Theseus_V3_rev4 (Autodesk Fusion 360 design; units mm, degrees)
Autodesk Fusion 360 part; units mm, degrees
note: some values were not read from the file. Chosen so that the rebuilt part matches the saved one: which bodies a step acts on; a direction. Set by a fixed rule: which sketch regions a step uses.
(part 1 of 5)
sketch "Tub shell sketch" plane through (0, 0, 0) normal (0, 0, 1) x (1, 0, 0) in component "Tub"
  circle A0 centre (0, 0) radius 105
extrude "Tub shell" add sketch "Tub shell sketch" along normal blind 52 from surface at 35 makes body 1 in component "Tub"
sketch "Cavity sketch" plane through (0, 0, 0) normal (0, 0, 1) x (1, 0, 0) in component "Tub"
  circle A0 centre (0, 0) radius 103
extrude "Cavity" cut sketch "Cavity sketch" along normal blind 53 from surface at 39 bodies 1 in component "Tub"
sketch "Rear chamfer sketch" plane through (0, 0, 0) normal (0, 1, 0) x (1, 0, 0) in component "Tub"
  line L0 (-65, -35) -> (-112, -56.15)
  line L1 (-112, -56.15) -> (-112, -29)
  line L2 (-112, -29) -> (-65, -29)
  line L3 (-65, -29) -> (-65, -35)
extrude "Rear chamfer" cut sketch "Rear chamfer sketch" along normal blind 220 from surface at -110 bodies 1 in component "Tub"
sketch "Wheel opening and arch L sketch" plane through (0, 0, 0) normal (0, 0, 1) x (1, 0, 0) in component "Tub"
  line L0 (-44, 69) -> (44, 69)
  line L1 (44, 69) -> (44, 108)
  line L2 (44, 108) -> (-44, 108)
  line L3 (-44, 108) -> (-44, 69)
extrude "Wheel opening and arch L" cut sketch "Wheel opening and arch L sketch" along normal blind 49 from surface at 34 bodies 1 in component "Tub"
sketch "Camera notch L sketch" plane through (0, 0, 0) normal (0, 0, 1) x (1, 0, 0) in component "Tub"
  line L0 (-11.9288, 69) -> (18.0712, 69)
  line L1 (18.0712, 69) -> (18.0712, 108)
  line L2 (18.0712, 108) -> (-11.9288, 108)
  line L3 (-11.9288, 108) -> (-11.9288, 69)
extrude "Camera notch L" cut sketch "Camera notch L sketch" along normal blind 6 from surface at 82 bodies 1 in component "Tub"
sketch "Motor seat L sketch" plane through (0, 0, 0) normal (0, 1, 0) x (1, 0, 0) in component "Tub"
  circle A0 centre (0, -40) radius 10.15
extrude "Motor seat L" cut sketch "Motor seat L sketch" along normal blind 51.5 from surface at 13 bodies 1 in component "Tub"
sketch "Shaft notch L sketch" plane through (0, 0, 0) normal (0, 1, 0) x (1, 0, 0) in component "Tub"
  line L0 (-3, -34.5) -> (3, -34.5)
  line L1 (3, -34.5) -> (3, -44.5)
  line L2 (3, -44.5) -> (-3, -44.5)
  line L3 (-3, -44.5) -> (-3, -34.5)
extrude "Shaft notch L" cut sketch "Shaft notch L sketch" along normal blind 4.5 from surface at 64.5 bodies 1 in component "Tub"
sketch "Plate slot L sketch" plane through (0, 0, 0) normal (0, 0, 1) x (1, 0, 0) in component "Tub"
  line L0 (-16, 60.5) -> (24.5, 60.5)
  line L1 (24.5, 60.5) -> (24.5, 64.5)
  line L2 (24.5, 64.5) -> (-16, 64.5)
  line L3 (-16, 64.5) -> (-16, 60.5)
extrude "Plate slot L" cut sketch "Plate slot L sketch" along normal blind 5 from surface at 34.5 bodies 1 in component "Tub"
sketch "Wheel opening and arch R sketch" plane through (0, 0, 0) normal (0, 0, 1) x (1, 0, 0) in component "Tub"
  line L0 (-44, -108) -> (44, -108)
  line L1 (44, -108) -> (44, -69)
  line L2 (44, -69) -> (-44, -69)
  line L3 (-44, -69) -> (-44, -108)
extrude "Wheel opening and arch R" cut sketch "Wheel opening and arch R sketch" along normal blind 49 from surface at 34 bodies 1 in component "Tub"
sketch "Camera notch R sketch" plane through (0, 0, 0) normal (0, 0, 1) x (1, 0, 0) in component "Tub"
  line L0 (-11.9288, -108) -> (18.0712, -108)
  line L1 (18.0712, -108) -> (18.0712, -69)
  line L2 (18.0712, -69) -> (-11.9288, -69)
  line L3 (-11.9288, -69) -> (-11.9288, -108)
extrude "Camera notch R" cut sketch "Camera notch R sketch" along normal blind 6 from surface at 82 bodies 1 in component "Tub"
sketch "Motor seat R sketch" plane through (0, 0, 0) normal (0, 1, 0) x (1, 0, 0) in component "Tub"
  circle A0 centre (0, -40) radius 10.15
extrude "Motor seat R" cut sketch "Motor seat R sketch" along normal blind 51.5 from surface at -64.5 bodies 1 in component "Tub"
sketch "Shaft notch R sketch" plane through (0, 0, 0) normal (0, 1, 0) x (1, 0, 0) in component "Tub"
  line L0 (-3, -34.5) -> (3, -34.5)
  line L1 (3, -34.5) -> (3, -44.5)
  line L2 (3, -44.5) -> (-3, -44.5)
  line L3 (-3, -44.5) -> (-3, -34.5)
extrude "Shaft notch R" cut sketch "Shaft notch R sketch" along normal blind 4.5 from surface at -69 bodies 1 in component "Tub"
sketch "Plate slot R sketch" plane through (0, 0, 0) normal (0, 0, 1) x (1, 0, 0) in component "Tub"
  line L0 (-16, -64.5) -> (24.5, -64.5)
  line L1 (24.5, -64.5) -> (24.5, -60.5)
  line L2 (24.5, -60.5) -> (-16, -60.5)
  line L3 (-16, -60.5) -> (-16, -64.5)
extrude "Plate slot R" cut sketch "Plate slot R sketch" along normal blind 5 from surface at 34.5 bodies 1 in component "Tub"
sketch "Omni wheel opening sketch" plane through (0, 0, 0) normal (0, 0, 1) x (1, 0, 0) in component "Tub"
  line L0 (36.5, -11.3) -> (101, -11.3)
  line L1 (101, -11.3) -> (101, 17.3)
  line L2 (101, 17.3) -> (36.5, 17.3)
  line L3 (36.5, 17.3) -> (36.5, -11.3)
extrude "Omni wheel opening" cut sketch "Omni wheel opening sketch" along normal blind 6 from surface at 34 bodies 1 in component "Tub"
sketch "Omni arm corridor sketch" plane through (0, 0, 0) normal (0, 0, 1) x (1, 0, 0) in component "Tub"
  line L0 (16.5928, 7.5) -> (80, 7.5)
  line L1 (80, 7.5) -> (80, 21)
  line L2 (80, 21) -> (16.5928, 21)
  line L3 (16.5928, 21) -> (16.5928, 7.5)
extrude "Omni arm corridor" cut sketch "Omni arm corridor sketch" along normal blind 6 from surface at 34 bodies 1 in component "Tub"
sketch "Omni pillar sketch" plane through (0, 0, 0) normal (0, 0, 1) x (1, 0, 0) in component "Tub"
  line L0 (17.7928, 3.5) -> (35.5, 3.5)
  line L1 (35.5, 3.5) -> (35.5, 7.5)
  line L2 (35.5, 7.5) -> (17.7928, 7.5)
  line L3 (17.7928, 7.5) -> (17.7928, 3.5)
extrude "Omni pillar" add sketch "Omni pillar sketch" along normal blind 11 from surface at 38.5 bodies 1 in component "Tub"
sketch "Omni pillar tail sketch" plane through (0, 0, 0) normal (0, 0, 1) x (1, 0, 0) in component "Tub"
  line L0 (9.8928, 3.5) -> (17.7928, 3.5)
  line L1 (17.7928, 3.5) -> (17.7928, 12)
  line L2 (17.7928, 12) -> (9.8928, 12)
  line L3 (9.8928, 12) -> (9.8928, 3.5)
extrude "Omni pillar tail" add sketch "Omni pillar tail sketch" along normal blind 5.5 from surface at 38.5 bodies 1 in component "Tub"
sketch "Omni ear sketch" plane through (0, 0, 0) normal (0, 0, 1) x (1, 0, 0) in component "Tub"
  line L0 (19.0928, 21) -> (36.5, 21)
  line L1 (36.5, 21) -> (36.5, 29.8)
  line L2 (36.5, 29.8) -> (19.0928, 29.8)
  line L3 (19.0928, 29.8) -> (19.0928, 21)
extrude "Omni ear" add sketch "Omni ear sketch" along normal blind 8.5 from surface at 38.5 bodies 1 in component "Tub"
sketch "Pivot hole pillar sketch" plane through (0, 0, 0) normal (0, 1, 0) x (1, 0, 0) in component "Tub"
  circle A0 centre (24.0928, -42) radius 1.6
extrude "Pivot hole pillar" cut sketch "Pivot hole pillar sketch" along normal blind 6 from surface at 2.5 bodies 1 in component "Tub"
sketch "Pivot thread hole ear sketch" plane through (0, 0, 0) normal (0, 1, 0) x (1, 0, 0) in component "Tub"
  circle A0 centre (24.0928, -42) radius 1.5
extrude "Pivot thread hole ear" cut sketch "Pivot thread hole ear sketch" along normal blind 8.1 from surface at 20.5 bodies 1 in component "Tub"
sketch "Stop hole pillar sketch" plane through (0, 0, 0) normal (0, 1, 0) x (1, 0, 0) in component "Tub"
  circle A0 centre (32.0923, -42.0904) radius 1.6
extrude "Stop hole pillar" cut sketch "Stop hole pillar sketch" along normal blind 6 from surface at 2.5 bodies 1 in component "Tub"
sketch "Stop thread hole ear sketch" plane through (0, 0, 0) normal (0, 1, 0) x (1, 0, 0) in component "Tub"
  circle A0 centre (32.0923, -42.0904) radius 1.5
extrude "Stop thread hole ear" cut sketch "Stop thread hole ear sketch" along normal blind 8.1 from surface at 20.5 bodies 1 in component "Tub"
sketch "Adjuster hole tail sketch" plane through (0, 0, 0) normal (0, 0, 1) x (1, 0, 0) in component "Tub"
  circle A0 centre (14.0928, 8.8) radius 1.5
extrude "Adjuster hole tail" cut sketch "Adjuster hole tail sketch" along normal blind 6.8 from surface at 38.2 bodies 1 in component "Tub"
sketch "Floor port FP hole sketch" plane through (0, 0, 0) normal (0, 0, 1) x (1, 0, 0) in component "Tub"
  line L0 (64.35, 24.35) -> (85.65, 24.35)
  line L1 (85.65, 24.35) -> (85.65, 45.65)
  line L2 (85.65, 45.65) -> (64.35, 45.65)
  line L3 (64.35, 45.65) -> (64.35, 24.35)
extrude "Floor port FP hole" cut sketch "Floor port FP hole sketch" along normal blind 6 from surface at 34 bodies 1 in component "Tub"
sketch "Silver module SM hole sketch" plane through (0, 0, 0) normal (0, 0, 1) x (1, 0, 0) in component "Tub"
  line L0 (64.5, -38.5) -> (85.5, -38.5)
  line L1 (85.5, -38.5) -> (85.5, -15.5)
  line L2 (85.5, -15.5) -> (64.5, -15.5)
  line L3 (64.5, -15.5) -> (64.5, -38.5)
extrude "Silver module SM hole" cut sketch "Silver module SM hole sketch" along normal blind 6 from surface at 34 bodies 1 in component "Tub"
sketch "Chute hole tool B left sketch" plane through (0, 0, 0) normal (0, 0, 1) x (1, 0, 0) in component "Tub"
  line L0 (-11.5, -10) -> (11.5, -10)
  line L1 (11.5, -10) -> (11.5, 13)
  line L2 (11.5, 13) -> (-11.5, 13)
  line L3 (-11.5, 13) -> (-11.5, -10)
extrude "Chute hole tool B left" add sketch "Chute hole tool B left sketch" along normal blind 79.2151 separate body makes body 2 in component "Tub"
move_body "Move1" bodies 2 to x (-0.977496, -0.210954, 0) y (-0.112564, 0.521586, 0.845741) z (-0.178413, 0.826708, -0.533594) at (-47.2943, 27.2943, 79.5) in component "Tub"
combine "Combine1" operation cut target body 1 tool bodies 2 in component "Tub"
sketch "Chute hole tool A right sketch" plane through (0, 0, 0) normal (0, 0, 1) x (1, 0, 0) in component "Tub"
  line L0 (-11.5, -10) -> (11.5, -10)
  line L1 (11.5, -10) -> (11.5, 13)
  line L2 (11.5, 13) -> (-11.5, 13)
  line L3 (-11.5, 13) -> (-11.5, -10)
extrude "Chute hole tool A right" add sketch "Chute hole tool A right sketch" along normal blind 79.2151 separate body makes body 3 in component "Tub"
move_body "Move2" bodies 3 to x (0.977496, -0.210954, 0) y (-0.112564, -0.521586, 0.845741) z (-0.178413, -0.826708, -0.533594) at (-47.2943, -27.2943, 79.5) in component "Tub"
combine "Combine2" operation cut target body 1 tool bodies 3 in component "Tub"
sketch "Bumper recess L sketch" plane through (0, 0, 0) normal (0, 0, 1) x (1, 0, 0) in component "Tub"
  arc A0 (106.949, 15.0307) -> (50.7029, 95.3583) centre (0, 0) ccw
  line L0 (50.7029, 95.3583) -> (48.5903, 91.3851)
  arc A1 (102.4927, 14.4044) -> (48.5903, 91.3851) centre (0, 0) ccw
  line L1 (102.4927, 14.4044) -> (106.949, 15.0307)
extrude "Bumper recess L" cut sketch "Bumper recess L sketch" along normal blind 25 from surface at 40 bodies 1 in component "Tub"
sketch "Bumper recess wall L sketch" plane through (0, 0, 0) normal (0, 0, 1) x (1, 0, 0) in component "Tub"
  arc A0 (102.1957, 14.3627) -> (48.4495, 91.1202) centre (0, 0) ccw
  line L0 (48.4495, 91.1202) -> (47.6514, 89.6192)
  arc A1 (100.5122, 14.1261) -> (47.6514, 89.6192) centre (0, 0) ccw
  line L1 (100.5122, 14.1261) -> (102.1957, 14.3627)
extrude "Bumper recess wall L" add sketch "Bumper recess wall L sketch" along normal blind 27 from surface at 39 bodies 1 in component "Tub"
sketch "Bumper switch pocket L sketch" plane through (0, 0, 0) normal (0, 0, 1) x (1, 0, 0) in component "Tub"
  line L0 (98.18, 21.6448) -> (101.576, 22.4916)
  line L1 (101.576, 22.4916) -> (100.2455, 27.8282)
  line L2 (100.2455, 27.8282) -> (96.8494, 26.9815)
  line L3 (96.8494, 26.9815) -> (98.18, 21.6448)
extrude "Bumper switch pocket L" cut sketch "Bumper switch pocket L sketch" along normal blind 12 from surface at 46.5 bodies 1 in component "Tub"
sketch "Bumper recess R sketch" plane through (0, 0, 0) normal (0, 0, 1) x (1, 0, 0) in component "Tub"
  arc A0 (50.7029, -95.3583) -> (106.949, -15.0307) centre (0, 0) ccw
  line L0 (106.949, -15.0307) -> (102.4927, -14.4044)
  arc A1 (48.5903, -91.3851) -> (102.4927, -14.4044) centre (0, 0) ccw
  line L1 (48.5903, -91.3851) -> (50.7029, -95.3583)
extrude "Bumper recess R" cut sketch "Bumper recess R sketch" along normal blind 25 from surface at 40 bodies 1 in component "Tub"
sketch "Bumper recess wall R sketch" plane through (0, 0, 0) normal (0, 0, 1) x (1, 0, 0) in component "Tub"
  arc A0 (48.4495, -91.1202) -> (102.1957, -14.3627) centre (0, 0) ccw
  line L0 (102.1957, -14.3627) -> (100.5122, -14.1261)
  arc A1 (47.6514, -89.6192) -> (100.5122, -14.1261) centre (0, 0) ccw
  line L1 (47.6514, -89.6192) -> (48.4495, -91.1202)
extrude "Bumper recess wall R" add sketch "Bumper recess wall R sketch" along normal blind 27 from surface at 39 bodies 1 in component "Tub"
sketch "Bumper switch pocket R sketch" plane through (0, 0, 0) normal (0, 0, 1) x (1, 0, 0) in component "Tub"
  line L0 (96.8494, -26.9815) -> (100.2455, -27.8282)
  line L1 (100.2455, -27.8282) -> (101.576, -22.4916)
  line L2 (101.576, -22.4916) -> (98.18, -21.6448)
  line L3 (98.18, -21.6448) -> (96.8494, -26.9815)
extrude "Bumper switch pocket R" cut sketch "Bumper switch pocket R sketch" along normal blind 12 from surface at 46.5 bodies 1 in component "Tub"
sketch "Insert boss +12 sketch" plane through (0, 0, 0) normal (0, 0, 1) x (1, 0, 0) in component "Tub"
  circle A0 centre (95.3694, 20.2714) radius 6
  line L0 (96.4089, 15.3807) -> (102.7669, 16.7321)
  line L1 (102.7669, 16.7321) -> (100.6878, 26.5136)
  line L2 (100.6878, 26.5136) -> (94.3298, 25.1621)
  line L3 (94.3298, 25.1621) -> (96.4089, 15.3807)
extrude "Insert boss +12" add sketch "Insert boss +12 sketch" along normal blind 10 from surface at 77 bodies 1 in component "Tub"
sketch "Insert boss +60 sketch" plane through (0, 0, 0) normal (0, 0, 1) x (1, 0, 0) in component "Tub"
  circle A0 centre (48.75, 84.4375) radius 6
  line L0 (53.0801, 81.9375) -> (56.3301, 87.5666)
  line L1 (56.3301, 87.5666) -> (47.6699, 92.5666)
  line L2 (47.6699, 92.5666) -> (44.4199, 86.9375)
  line L3 (44.4199, 86.9375) -> (53.0801, 81.9375)
extrude "Insert boss +60" add sketch "Insert boss +60 sketch" along normal blind 10 from surface at 77 bodies 1 in component "Tub"
sketch "Insert boss +118 sketch" plane through (0, 0, 0) normal (0, 0, 1) x (1, 0, 0) in component "Tub"
  circle A0 centre (-45.7735, 86.0874) radius 6
  line L0 (-41.3587, 88.4347) -> (-44.4103, 94.1739)
  line L1 (-44.4103, 94.1739) -> (-53.2398, 89.4792)
  line L2 (-53.2398, 89.4792) -> (-50.1882, 83.74)
  line L3 (-50.1882, 83.74) -> (-41.3587, 88.4347)
extrude "Insert boss +118" add sketch "Insert boss +118 sketch" along normal blind 10 from surface at 77 bodies 1 in component "Tub"
sketch "Insert boss -12 sketch" plane through (0, 0, 0) normal (0, 0, 1) x (1, 0, 0) in component "Tub"
  circle A0 centre (95.3694, -20.2714) radius 6
  line L0 (94.3298, -25.1621) -> (100.6878, -26.5136)
  line L1 (100.6878, -26.5136) -> (102.7669, -16.7321)
  line L2 (102.7669, -16.7321) -> (96.4089, -15.3807)
  line L3 (96.4089, -15.3807) -> (94.3298, -25.1621)
extrude "Insert boss -12" add sketch "Insert boss -12 sketch" along normal blind 10 from surface at 77 bodies 1 in component "Tub"
sketch "Insert boss -60 sketch" plane through (0, 0, 0) normal (0, 0, 1) x (1, 0, 0) in component "Tub"
  circle A0 centre (48.75, -84.4375) radius 6
  line L0 (44.4199, -86.9375) -> (47.6699, -92.5666)
  line L1 (47.6699, -92.5666) -> (56.3301, -87.5666)
  line L2 (56.3301, -87.5666) -> (53.0801, -81.9375)
  line L3 (53.0801, -81.9375) -> (44.4199, -86.9375)
extrude "Insert boss -60" add sketch "Insert boss -60 sketch" along normal blind 10 from surface at 77 bodies 1 in component "Tub"
sketch "Insert boss -118 sketch" plane through (0, 0, 0) normal (0, 0, 1) x (1, 0, 0) in component "Tub"
  circle A0 centre (-45.7735, -86.0874) radius 6
  line L0 (-50.1882, -83.74) -> (-53.2398, -89.4792)
  line L1 (-53.2398, -89.4792) -> (-44.4103, -94.1739)
  line L2 (-44.4103, -94.1739) -> (-41.3587, -88.4347)
  line L3 (-41.3587, -88.4347) -> (-50.1882, -83.74)
extrude "Insert boss -118" add sketch "Insert boss -118 sketch" along normal blind 10 from surface at 77 bodies 1 in component "Tub"
sketch "Cradle web rear L sketch" plane through (0, 0, 0) normal (0, 1, 0) x (1, 0, 0) in component "Tub"
  line L0 (-16, -38.5) -> (-3, -38.5)
  line L1 (-3, -38.5) -> (-3, -52)
  line L2 (-3, -52) -> (-16, -52)
  line L3 (-16, -52) -> (-16, -38.5)
extrude "Cradle web rear L" add sketch "Cradle web rear L sketch" along normal blind 2.5 from surface at 64.5 bodies 1 in component "Tub"
sketch "Cradle web front L sketch" plane through (0, 0, 0) normal (0, 1, 0) x (1, 0, 0) in component "Tub"
  line L0 (3, -38.5) -> (27.5, -38.5)
  line L1 (27.5, -38.5) -> (27.5, -52)
  line L2 (27.5, -52) -> (3, -52)
  line L3 (3, -52) -> (3, -38.5)
extrude "Cradle web front L" add sketch "Cradle web front L sketch" along normal blind 2.5 from surface at 64.5 bodies 1 in component "Tub"
sketch "Cradle ledge front L sketch" plane through (0, 0, 0) normal (0, 1, 0) x (1, 0, 0) in component "Tub"
  line L0 (10.6, -38.5) -> (27.5, -38.5)
  line L1 (27.5, -38.5) -> (27.5, -49)
  line L2 (27.5, -49) -> (10.6, -49)
  line L3 (10.6, -49) -> (10.6, -38.5)
extrude "Cradle ledge front L" add sketch "Cradle ledge front L sketch" along normal blind 4 from surface at 56.5 bodies 1 in component "Tub"
sketch "Cradle ledge rear L sketch" plane through (0, 0, 0) normal (0, 1, 0) x (1, 0, 0) in component "Tub"
  line L0 (-16, -38.5) -> (-10.6, -38.5)
  line L1 (-10.6, -38.5) -> (-10.6, -49)
  line L2 (-10.6, -49) -> (-16, -49)
  line L3 (-16, -49) -> (-16, -38.5)
extrude "Cradle ledge rear L" add sketch "Cradle ledge rear L sketch" along normal blind 4 from surface at 56.5 bodies 1 in component "Tub"
sketch "Cradle prong front L sketch" plane through (0, 0, 0) normal (0, 1, 0) x (1, 0, 0) in component "Tub"
  line L0 (13, -38.5) -> (13, -48)
  line L1 (13, -48) -> (8, -48)
  line L2 (8, -48) -> (7.8607, -46.5)
  line L3 (7.8607, -46.5) -> (8.544, -45.5714)
  line L4 (8.544, -45.5714) -> (9.0821, -44.6429)
  line L5 (9.0821, -44.6429) -> (9.4997, -43.7143)
  line L6 (9.4997, -43.7143) -> (9.8122, -42.7857)
  line L7 (9.8122, -42.7857) -> (10.0295, -41.8571)
  line L8 (10.0295, -41.8571) -> (10.1576, -40.9286)
  line L9 (10.1576, -40.9286) -> (10.2, -40)
  line L10 (10.2, -40) -> (10.6, -38.5)
  line L11 (10.6, -38.5) -> (13, -38.5)
extrude "Cradle prong front L" add sketch "Cradle prong front L sketch" along normal blind 32 from surface at 28.5 separate body makes body 4 in component "Tub"
sketch "Cradle prong rear L sketch" plane through (0, 0, 0) normal (0, 1, 0) x (1, 0, 0) in component "Tub"
  line L0 (-13, -38.5) -> (-13, -48)
  line L1 (-13, -48) -> (-8, -48)
  line L2 (-8, -48) -> (-7.8607, -46.5)
  line L3 (-7.8607, -46.5) -> (-8.544, -45.5714)
  line L4 (-8.544, -45.5714) -> (-9.0821, -44.6429)
  line L5 (-9.0821, -44.6429) -> (-9.4997, -43.7143)
  line L6 (-9.4997, -43.7143) -> (-9.8122, -42.7857)
  line L7 (-9.8122, -42.7857) -> (-10.0295, -41.8571)
  line L8 (-10.0295, -41.8571) -> (-10.1576, -40.9286)
  line L9 (-10.1576, -40.9286) -> (-10.2, -40)
  line L10 (-10.2, -40) -> (-10.6, -38.5)
  line L11 (-10.6, -38.5) -> (-13, -38.5)
extrude "Cradle prong rear L" add sketch "Cradle prong rear L sketch" along normal blind 32 from surface at 28.5 separate body makes body 5 in component "Tub"
sketch "Cradle web rear R sketch" plane through (0, 0, 0) normal (0, 1, 0) x (1, 0, 0) in component "Tub"
  line L0 (-16, -38.5) -> (-3, -38.5)
  line L1 (-3, -38.5) -> (-3, -52)
  line L2 (-3, -52) -> (-16, -52)
  line L3 (-16, -52) -> (-16, -38.5)
extrude "Cradle web rear R" add sketch "Cradle web rear R sketch" along normal blind 2.5 from surface at -67 bodies 1 in component "Tub"
sketch "Cradle web front R sketch" plane through (0, 0, 0) normal (0, 1, 0) x (1, 0, 0) in component "Tub"
  line L0 (3, -38.5) -> (27.5, -38.5)
  line L1 (27.5, -38.5) -> (27.5, -52)
  line L2 (27.5, -52) -> (3, -52)
  line L3 (3, -52) -> (3, -38.5)
extrude "Cradle web front R" add sketch "Cradle web front R sketch" along normal blind 2.5 from surface at -67 bodies 1 in component "Tub"
sketch "Cradle ledge front R sketch" plane through (0, 0, 0) normal (0, 1, 0) x (1, 0, 0) in component "Tub"
  line L0 (10.6, -38.5) -> (27.5, -38.5)
  line L1 (27.5, -38.5) -> (27.5, -49)
  line L2 (27.5, -49) -> (10.6, -49)
  line L3 (10.6, -49) -> (10.6, -38.5)
extrude "Cradle ledge front R" add sketch "Cradle ledge front R sketch" along normal blind 4 from surface at -60.5 bodies 1 in component "Tub"
sketch "Cradle ledge rear R sketch" plane through (0, 0, 0) normal (0, 1, 0) x (1, 0, 0) in component "Tub"
  line L0 (-16, -38.5) -> (-10.6, -38.5)
  line L1 (-10.6, -38.5) -> (-10.6, -49)
  line L2 (-10.6, -49) -> (-16, -49)
  line L3 (-16, -49) -> (-16, -38.5)
extrude "Cradle ledge rear R" add sketch "Cradle ledge rear R sketch" along normal blind 4 from surface at -60.5 bodies 1 in component "Tub"
sketch "Cradle prong front R sketch" plane through (0, 0, 0) normal (0, 1, 0) x (1, 0, 0) in component "Tub"
  line L0 (13, -38.5) -> (13, -48)
  line L1 (13, -48) -> (8, -48)
  line L2 (8, -48) -> (7.8607, -46.5)
  line L3 (7.8607, -46.5) -> (8.544, -45.5714)
  line L4 (8.544, -45.5714) -> (9.0821, -44.6429)
  line L5 (9.0821, -44.6429) -> (9.4997, -43.7143)
  line L6 (9.4997, -43.7143) -> (9.8122, -42.7857)
  line L7 (9.8122, -42.7857) -> (10.0295, -41.8571)
  line L8 (10.0295, -41.8571) -> (10.1576, -40.9286)
  line L9 (10.1576, -40.9286) -> (10.2, -40)
  line L10 (10.2, -40) -> (10.6, -38.5)
  line L11 (10.6, -38.5) -> (13, -38.5)
extrude "Cradle prong front R" add sketch "Cradle prong front R sketch" along normal blind 32 from surface at -60.5 separate body makes body 6 in component "Tub"
sketch "Cradle prong rear R sketch" plane through (0, 0, 0) normal (0, 1, 0) x (1, 0, 0) in component "Tub"
  line L0 (-13, -38.5) -> (-13, -48)
  line L1 (-13, -48) -> (-8, -48)
  line L2 (-8, -48) -> (-7.8607, -46.5)
  line L3 (-7.8607, -46.5) -> (-8.544, -45.5714)
  line L4 (-8.544, -45.5714) -> (-9.0821, -44.6429)
  line L5 (-9.0821, -44.6429) -> (-9.4997, -43.7143)
  line L6 (-9.4997, -43.7143) -> (-9.8122, -42.7857)
  line L7 (-9.8122, -42.7857) -> (-10.0295, -41.8571)
  line L8 (-10.0295, -41.8571) -> (-10.1576, -40.9286)
  line L9 (-10.1576, -40.9286) -> (-10.2, -40)
  line L10 (-10.2, -40) -> (-10.6, -38.5)
  line L11 (-10.6, -38.5) -> (-13, -38.5)
extrude "Cradle prong rear R" add sketch "Cradle prong rear R sketch" along normal blind 32 from surface at -60.5 separate body makes body 7 in component "Tub"
sketch "Tray leg sketch" plane through (0, 0, 0) normal (0, 0, 1) x (1, 0, 0) in component "Tub"
  circle A0 centre (66.4605, 60.5271) radius 3
extrude "Tray leg" add sketch "Tray leg sketch" along normal blind 11 from surface at 38.5 bodies 1 in component "Tub"
sketch "Tray leg sketch (1)" plane through (0, 0, 0) normal (0, 0, 1) x (1, 0, 0) in component "Tub"
  circle A0 centre (49.3095, 31.1019) radius 3
extrude "Tray leg (1)" add sketch "Tray leg sketch (1)" along normal blind 11 from surface at 38.5 bodies 1 in component "Tub"
sketch "Tray leg sketch (2)" plane through (0, 0, 0) normal (0, 0, 1) x (1, 0, 0) in component "Tub"
  circle A0 centre (32.7439, 44.4277) radius 3
extrude "Tray leg (2)" add sketch "Tray leg sketch (2)" along normal blind 11 from surface at 38.5 bodies 1 in component "Tub"
sketch "Battery tray sketch" plane through (0, 0, 0) normal (0, 0, 1) x (1, 0, 0) in component "Tub"
  line L0 (6.7594, 19.0297) -> (77.6656, 31.5324)
  line L1 (77.6656, 31.5324) -> (71.2406, 67.9703)
  line L2 (71.2406, 67.9703) -> (0.3344, 55.4676)
  line L3 (0.3344, 55.4676) -> (6.7594, 19.0297)
extrude "Battery tray" add sketch "Battery tray sketch" along normal blind 2 from surface at 49 bodies 1 in component "Tub"
sketch "Battery stop sketch" plane through (0, 0, 0) normal (0, 0, 1) x (1, 0, 0) in component "Tub"
  line L0 (77.1732, 31.4456) -> (79.1428, 31.7929)
  line L1 (79.1428, 31.7929) -> (72.7178, 68.2308)
  line L2 (72.7178, 68.2308) -> (70.7482, 67.8835)
  line L3 (70.7482, 67.8835) -> (77.1732, 31.4456)
extrude "Battery stop" add sketch "Battery stop sketch" along normal blind 6.5 from surface at 50.5 bodies 1 in component "Tub"
sketch "Battery tray notch sketch" plane through (0, 0, 0) normal (0, 0, 1) x (1, 0, 0) in component "Tub"
  line L0 (-12, 13) -> (12, 13)
  line L1 (12, 13) -> (12, 62)
  line L2 (12, 62) -> (-12, 62)
  line L3 (-12, 62) -> (-12, 13)
extrude "Battery tray notch" cut sketch "Battery tray notch sketch" along normal blind 4 from surface at 48 bodies 1 in component "Tub"
sketch "Insert hole +12 sketch" plane through (0, 0, 0) normal (0, 0, 1) x (1, 0, 0) in component "Tub"
  circle A0 centre (95.3694, 20.2714) radius 2
extrude "Insert hole +12" cut sketch "Insert hole +12 sketch" along normal blind 7 from surface at 81 bodies 1 in component "Tub"
sketch "Insert hole +60 sketch" plane through (0, 0, 0) normal (0, 0, 1) x (1, 0, 0) in component "Tub"
  circle A0 centre (48.75, 84.4375) radius 2
extrude "Insert hole +60" cut sketch "Insert hole +60 sketch" along normal blind 7 from surface at 81 bodies 1 in component "Tub"
sketch "Insert hole +118 sketch" plane through (0, 0, 0) normal (0, 0, 1) x (1, 0, 0) in component "Tub"
  circle A0 centre (-45.7735, 86.0874) radius 2
extrude "Insert hole +118" cut sketch "Insert hole +118 sketch" along normal blind 7 from surface at 81 bodies 1 in component "Tub"
sketch "Insert hole -12 sketch" plane through (0, 0, 0) normal (0, 0, 1) x (1, 0, 0) in component "Tub"
  circle A0 centre (95.3694, -20.2714) radius 2
extrude "Insert hole -12" cut sketch "Insert hole -12 sketch" along normal blind 7 from surface at 81 bodies 1 in component "Tub"
sketch "Insert hole -60 sketch" plane through (0, 0, 0) normal (0, 0, 1) x (1, 0, 0) in component "Tub"
  circle A0 centre (48.75, -84.4375) radius 2
extrude "Insert hole -60" cut sketch "Insert hole -60 sketch" along normal blind 7 from surface at 81 bodies 1 in component "Tub"
sketch "Insert hole -118 sketch" plane through (0, 0, 0) normal (0, 0, 1) x (1, 0, 0) in component "Tub"
  circle A0 centre (-45.7735, -86.0874) radius 2
extrude "Insert hole -118" cut sketch "Insert hole -118 sketch" along normal blind 7 from surface at 81 bodies 1 in component "Tub"
sketch "IMU posts sketch" plane through (0, 0, 0) normal (0, 0, 1) x (1, 0, 0) in component "Tub"
  line L0 (-42.5, 3.5) -> (-37.5, 3.5)
  line L1 (-37.5, 3.5) -> (-37.5, 8.5)
  line L2 (-37.5, 8.5) -> (-42.5, 8.5)
  line L3 (-42.5, 8.5) -> (-42.5, 3.5)
  line L4 (-42.5, -8.5) -> (-37.5, -8.5)
  line L5 (-37.5, -8.5) -> (-37.5, -3.5)
  line L6 (-37.5, -3.5) -> (-42.5, -3.5)
  line L7 (-42.5, -3.5) -> (-42.5, -8.5)
  line L8 (-62.5, 3.5) -> (-57.5, 3.5)
  line L9 (-57.5, 3.5) -> (-57.5, 8.5)
  line L10 (-57.5, 8.5) -> (-62.5, 8.5)
  line L11 (-62.5, 8.5) -> (-62.5, 3.5)
  line L12 (-62.5, -8.5) -> (-57.5, -8.5)
  line L13 (-57.5, -8.5) -> (-57.5, -3.5)
  line L14 (-57.5, -3.5) -> (-62.5, -3.5)
  line L15 (-62.5, -3.5) -> (-62.5, -8.5)
extrude "IMU posts" add sketch "IMU posts sketch" along normal blind 5.5 from surface at 38.5 bodies 1 in component "Tub"
sketch "IMU post pilots sketch" plane through (0, 0, 0) normal (0, 0, 1) x (1, 0, 0) in component "Tub"
  line L0 (-41, 5) -> (-39, 5)
  line L1 (-39, 5) -> (-39, 7)
  line L2 (-39, 7) -> (-41, 7)
  line L3 (-41, 7) -> (-41, 5)
  line L4 (-41, -7) -> (-39, -7)
  line L5 (-39, -7) -> (-39, -5)
  line L6 (-39, -5) -> (-41, -5)
  line L7 (-41, -5) -> (-41, -7)
  line L8 (-61, 5) -> (-59, 5)
  line L9 (-59, 5) -> (-59, 7)
  line L10 (-59, 7) -> (-61, 7)
  line L11 (-61, 7) -> (-61, 5)
  line L12 (-61, -7) -> (-59, -7)
  line L13 (-59, -7) -> (-59, -5)
  line L14 (-59, -5) -> (-61, -5)
  line L15 (-61, -5) -> (-61, -7)
extrude "IMU post pilots" cut sketch "IMU post pilots sketch" along normal blind 5.5 from surface at 39.5 bodies 1 in component "Tub"
sketch "USB-C socket hole sketch" plane through (0, 0, 0) normal (0, 0, 1) x (1, 0, 0) in component "Tub"
  line L0 (87.5938, -46.6617) -> (95.8158, -50.3224)
  line L1 (95.8158, -50.3224) -> (101.5101, -37.5327)
  line L2 (101.5101, -37.5327) -> (93.2882, -33.8721)
  line L3 (93.2882, -33.8721) -> (87.5938, -46.6617)
extrude "USB-C socket hole" cut sketch "USB-C socket hole sketch" along normal blind 8 from surface at 71 bodies 1 in component "Tub"
sketch "Wheel L sketch" plane through (0, 0, 0) normal (0, 1, 0) x (1, 0, 0) in component "Wheel L"
  circle A0 centre (0, -40) radius 40
extrude "Wheel L" add sketch "Wheel L sketch" along normal blind 20 from surface at 70 separate body makes body 8 in component "Wheel L"
sketch "Shaft bore sketch" plane through (0, 0, 0) normal (0, 1, 0) x (1, 0, 0) in component "Wheel L"
  circle A0 centre (0, -40) radius 1.5
extrude "Shaft bore" cut sketch "Shaft bore sketch" along normal blind 22 from surface at 69 bodies 8 in component "Wheel L"
sketch "Encoder L sketch" plane through (0, 0, 0) normal (0, 1, 0) x (1, 0, 0) in component "Motor L"
  circle A0 centre (0, -40) radius 9
extrude "Encoder L" add sketch "Encoder L sketch" along normal blind 3 from surface at 14 separate body makes body 9 in component "Motor L"
sketch "Gearmotor L sketch" plane through (0, 0, 0) normal (0, 1, 0) x (1, 0, 0) in component "Motor L"
  circle A0 centre (0, -40) radius 10
extrude "Gearmotor L" add sketch "Gearmotor L sketch" along normal blind 44 from surface at 17 separate body makes body 10 in component "Motor L"
sketch "Motor shaft L sketch" plane through (0, 0, 0) normal (0, 1, 0) x (1, 0, 0) in component "Motor L"
  circle A0 centre (0, -40) radius 1.5
extrude "Motor shaft L" add sketch "Motor shaft L sketch" along normal blind 19 from surface at 61 separate body makes body 11 in component "Motor L"
sketch "Wheel R sketch" plane through (0, 0, 0) normal (0, 1, 0) x (1, 0, 0) in component "Wheel R"
  circle A0 centre (0, -40) radius 40
extrude "Wheel R" add sketch "Wheel R sketch" along normal blind 20 from surface at -90 separate body makes body 12 in component "Wheel R"
sketch "Shaft bore sketch (2)" plane through (0, 0, 0) normal (0, 1, 0) x (1, 0, 0) in component "Wheel R"
  circle A0 centre (0, -40) radius 1.5
extrude "Shaft bore'" cut sketch "Shaft bore sketch (2)" along normal blind 22 from surface at -91 bodies 12 in component "Wheel R"
sketch "Encoder R sketch" plane through (0, 0, 0) normal (0, 1, 0) x (1, 0, 0) in component "Motor R"
  circle A0 centre (0, -40) radius 9
extrude "Encoder R" add sketch "Encoder R sketch" along normal blind 3 from surface at -17 separate body makes body 13 in component "Motor R"
sketch "Gearmotor R sketch" plane through (0, 0, 0) normal (0, 1, 0) x (1, 0, 0) in component "Motor R"
  circle A0 centre (0, -40) radius 10
extrude "Gearmotor R" add sketch "Gearmotor R sketch" along normal blind 44 from surface at -61 separate body makes body 14 in component "Motor R"
sketch "Motor shaft R sketch" plane through (0, 0, 0) normal (0, 1, 0) x (1, 0, 0) in component "Motor R"
  circle A0 centre (0, -40) radius 1.5
extrude "Motor shaft R" add sketch "Motor shaft R sketch" along normal blind 19 from surface at -80 separate body makes body 15 in component "Motor R"
sketch "Face plate L sketch" plane through (0, 0, 0) normal (0, 1, 0) x (1, 0, 0) in component "Face plate L"
  line L0 (-15.5, -35.5) -> (23.5, -35.5)
  line L1 (23.5, -35.5) -> (23.5, -46)
  line L2 (23.5, -46) -> (15.5, -46)
  line L3 (15.5, -46) -> (15.5, -51)
  line L4 (15.5, -51) -> (-15.5, -51)
  line L5 (-15.5, -51) -> (-15.5, -35.5)
extrude "Face plate L" add sketch "Face plate L sketch" along normal blind 3 from surface at 61 separate body makes body 16 in component "Face plate L"
sketch "Shaft bore sketch (3)" plane through (0, 0, 0) normal (0, 1, 0) x (1, 0, 0) in component "Face plate L"
  circle A0 centre (0, -40) radius 2.2
extrude "Shaft bore''" cut sketch "Shaft bore sketch (3)" along normal blind 5 from surface at 60 bodies 16 in component "Face plate L"
sketch "Face plate R sketch" plane through (0, 0, 0) normal (0, 1, 0) x (1, 0, 0) in component "Face plate R"
  line L0 (-15.5, -35.5) -> (23.5, -35.5)
  line L1 (23.5, -35.5) -> (23.5, -46)
  line L2 (23.5, -46) -> (15.5, -46)
  line L3 (15.5, -46) -> (15.5, -51)
  line L4 (15.5, -51) -> (-15.5, -51)
  line L5 (-15.5, -51) -> (-15.5, -35.5)
extrude "Face plate R" add sketch "Face plate R sketch" along normal blind 3 from surface at -64 separate body makes body 17 in component "Face plate R"
sketch "Shaft bore sketch (4)" plane through (0, 0, 0) normal (0, 1, 0) x (1, 0, 0) in component "Face plate R"
  circle A0 centre (0, -40) radius 2.2
extrude "Shaft bore'''" cut sketch "Shaft bore sketch (4)" along normal blind 5 from surface at -65 bodies 17 in component "Face plate R"
sketch "Omni wheel sketch" plane through (0, 0, 0) normal (0, 1, 0) x (1, 0, 0) in component "Omni wheel"
  circle A0 centre (68.5, -30) radius 30
extrude "Omni wheel" add sketch "Omni wheel sketch" along normal blind 25.6 from surface at -9.8 separate body makes body 18 in component "Omni wheel"
sketch "Wheel bore sketch" plane through (0, 0, 0) normal (0, 1, 0) x (1, 0, 0) in component "Omni wheel"
  circle A0 centre (68.5, -30) radius 6
extrude "Wheel bore" cut sketch "Wheel bore sketch" along normal blind 27.6 from surface at -10.8 bodies 18 in component "Omni wheel"
sketch "Bearing inboard sketch" plane through (0, 0, 0) normal (0, 1, 0) x (1, 0, 0) in component "Omni wheel"
  circle A0 centre (68.5, -30) radius 6
  circle A1 centre (68.5, -30) radius 2
extrude "Bearing inboard" add sketch "Bearing inboard sketch" along normal blind 4 from surface at -4.8 separate body makes body 19 in component "Omni wheel"
sketch "Bearing outboard sketch" plane through (0, 0, 0) normal (0, 1, 0) x (1, 0, 0) in component "Omni wheel"
  circle A0 centre (68.5, -30) radius 6
  circle A1 centre (68.5, -30) radius 2
extrude "Bearing outboard" add sketch "Bearing outboard sketch" along normal blind 4 from surface at 11.8 separate body makes body 20 in component "Omni wheel"
sketch "Axle sleeve sketch" plane through (0, 0, 0) normal (0, 1, 0) x (1, 0, 0) in component "Omni wheel"
  circle A0 centre (68.5, -30) radius 3
  circle A1 centre (68.5, -30) radius 2.05
extrude "Axle sleeve" add sketch "Axle sleeve sketch" along normal blind 12.6 from surface at -0.8 separate body makes body 21 in component "Omni wheel"
sketch "Axle spacer sketch" plane through (0, 0, 0) normal (0, 1, 0) x (1, 0, 0) in component "Omni wheel"
  circle A0 centre (68.5, -30) radius 3
  circle A1 centre (68.5, -30) radius 2.05
extrude "Axle spacer" add sketch "Axle spacer sketch" along normal blind 1 from surface at 15.8 separate body makes body 22 in component "Omni wheel"
sketch "Arm bar sketch" plane through (0, 0, 0) normal (0, 1, 0) x (1, 0, 0) in component "Omni arm"
  line L0 (25.658, -47.7922) -> (70.0652, -35.7922)
  arc A0 (70.0652, -35.7922) -> (66.9348, -24.2078) centre (68.5, -30) ccw
  line L1 (66.9348, -24.2078) -> (22.5276, -36.2078)
  arc A1 (22.5276, -36.2078) -> (25.658, -47.7922) centre (24.0928, -42) ccw
extrude "Arm bar" add sketch "Arm bar sketch" along normal blind 3 from surface at 16.8 separate body makes body 23 in component "Omni arm"
sketch "Pivot bore sketch" plane through (0, 0, 0) normal (0, 1, 0) x (1, 0, 0) in component "Omni arm"
  circle A0 centre (24.0928, -42) radius 2.525
extrude "Pivot bore" cut sketch "Pivot bore sketch" along normal blind 5 from surface at 15.8 bodies 23 in component "Omni arm"
sketch "Axle hole sketch" plane through (0, 0, 0) normal (0, 1, 0) x (1, 0, 0) in component "Omni arm"
  circle A0 centre (68.5, -30) radius 2
extrude "Axle hole" cut sketch "Axle hole sketch" along normal blind 5 from surface at 15.8 bodies 23 in component "Omni arm"
sketch "Stop slot sketch" plane through (0, 0, 0) normal (0, 1, 0) x (1, 0, 0) in component "Omni arm"
  line L0 (32.3428, -36.994) -> (32.6114, -37.4662)
  line L1 (32.6114, -37.4662) -> (32.853, -37.9526)
  line L2 (32.853, -37.9526) -> (33.0668, -38.4519)
  line L3 (33.0668, -38.4519) -> (33.2523, -38.9625)
  line L4 (33.2523, -38.9625) -> (33.4087, -39.4826)
  line L5 (33.4087, -39.4826) -> (33.5355, -40.0107)
  line L6 (33.5355, -40.0107) -> (33.6325, -40.5452)
  line L7 (33.6325, -40.5452) -> (33.6992, -41.0842)
  line L8 (33.6992, -41.0842) -> (33.7355, -41.6262)
  line L9 (33.7355, -41.6262) -> (33.7413, -42.1693)
  line L10 (33.7413, -42.1693) -> (33.6047, -42.7984)
  line L11 (33.6047, -42.7984) -> (33.2376, -43.3274)
  line L12 (33.2376, -43.3274) -> (32.6961, -43.6756)
  line L13 (32.6961, -43.6756) -> (32.0626, -43.7901)
  line L14 (32.0626, -43.7901) -> (31.4335, -43.6534)
  line L15 (31.4335, -43.6534) -> (30.9045, -43.2864)
  line L16 (30.9045, -43.2864) -> (30.5563, -42.7449)
  line L17 (30.5563, -42.7449) -> (30.4418, -42.1114)
  line L18 (30.4418, -42.1114) -> (30.438, -41.754)
  line L19 (30.438, -41.754) -> (30.4141, -41.3974)
  line L20 (30.4141, -41.3974) -> (30.3702, -41.0427)
  line L21 (30.3702, -41.0427) -> (30.3064, -40.691)
  line L22 (30.3064, -40.691) -> (30.2229, -40.3435)
  line L23 (30.2229, -40.3435) -> (30.12, -40.0012)
  line L24 (30.12, -40.0012) -> (29.998, -39.6653)
  line L25 (29.998, -39.6653) -> (29.8573, -39.3367)
  line L26 (29.8573, -39.3367) -> (29.6983, -39.0166)
  line L27 (29.6983, -39.0166) -> (29.5216, -38.7059)
  line L28 (29.5216, -38.7059) -> (29.3014, -38.1009)
  line L29 (29.3014, -38.1009) -> (29.3295, -37.4578)
  line L30 (29.3295, -37.4578) -> (29.6016, -36.8743)
  line L31 (29.6016, -36.8743) -> (30.0763, -36.4394)
  line L32 (30.0763, -36.4394) -> (30.6812, -36.2192)
  line L33 (30.6812, -36.2192) -> (31.3244, -36.2473)
  line L34 (31.3244, -36.2473) -> (31.9079, -36.5194)
  line L35 (31.9079, -36.5194) -> (32.3428, -36.994)
extrude "Stop slot" cut sketch "Stop slot sketch" along normal blind 5 from surface at 15.8 bodies 23 in component "Omni arm"
sketch "Seat hole sketch" plane through (0, 0, 0) normal (0, 1, 0) x (1, 0, 0) in component "Omni arm"
  circle A0 centre (35.75, -42.9721) radius 1
extrude "Seat hole" cut sketch "Seat hole sketch" along normal blind 5 from surface at 15.8 bodies 23 in component "Omni arm"
sketch "Seat pin sketch" plane through (0, 0, 0) normal (0, 1, 0) x (1, 0, 0) in component "Omni arm"
  circle A0 centre (35.75, -42.9721) radius 1
extrude "Seat pin" add sketch "Seat pin sketch" along normal blind 6 from surface at 13.3 separate body makes body 24 in component "Omni arm"
sketch "Spring forward leg sketch" plane through (0, 0, 0) normal (0, 1, 0) x (1, 0, 0) in component "Omni arm"
  line L0 (29.7706, -45.1642) -> (37.0494, -43.7333)
  line L1 (37.0494, -43.7333) -> (37.358, -45.3033)
  line L2 (37.358, -45.3033) -> (30.0793, -46.7342)
  line L3 (30.0793, -46.7342) -> (29.7706, -45.1642)
extrude "Spring forward leg" add sketch "Spring forward leg sketch" along normal blind 1.6 from surface at 14.512 separate body makes body 25 in component "Omni arm"
sketch "Axle screw sketch" plane through (0, 0, 0) normal (0, 1, 0) x (1, 0, 0) in component "Omni pins"
  circle A0 centre (68.5, -30) radius 2
extrude "Axle screw" add sketch "Axle screw sketch" along normal blind 25 from surface at -5.3 separate body makes body 26 in component "Omni pins"
sketch "Axle screw head sketch" plane through (0, 0, 0) normal (0, 1, 0) x (1, 0, 0) in component "Omni pins"
  circle A0 centre (68.5, -30) radius 3.5
extrude "Axle screw head" add sketch "Axle screw head sketch" along normal blind 4 from surface at -9.3 separate body makes body 27 in component "Omni pins"
sketch "Axle washer sketch" plane through (0, 0, 0) normal (0, 1, 0) x (1, 0, 0) in component "Omni pins"
  circle A0 centre (68.5, -30) radius 3
  circle A1 centre (68.5, -30) radius 2.05
extrude "Axle washer" add sketch "Axle washer sketch" along normal blind 0.5 from surface at -5.3 separate body makes body 28 in component "Omni pins"
sketch "Pivot screw sketch" plane through (0, 0, 0) normal (0, 1, 0) x (1, 0, 0) in component "Omni pivot"
  circle A0 centre (24.0928, -42) radius 1.5
extrude "Pivot screw" add sketch "Pivot screw sketch" along normal blind 25 from surface at 3.5 separate body makes body 29 in component "Omni pivot"
sketch "Pivot screw head sketch" plane through (0, 0, 0) normal (0, 1, 0) x (1, 0, 0) in component "Omni pivot"
  circle A0 centre (24.0928, -42) radius 2.75
extrude "Pivot screw head" add sketch "Pivot screw head sketch" along normal blind 3 from surface at 0.5 separate body makes body 30 in component "Omni pivot"
sketch "Stop screw sketch" plane through (0, 0, 0) normal (0, 1, 0) x (1, 0, 0) in component "Omni pivot"
  circle A0 centre (32.0923, -42.0904) radius 1.5
extrude "Stop screw" add sketch "Stop screw sketch" along normal blind 25 from surface at 3.5 separate body makes body 31 in component "Omni pivot"
sketch "Stop screw head sketch" plane through (0, 0, 0) normal (0, 1, 0) x (1, 0, 0) in component "Omni pivot"
  circle A0 centre (32.0923, -42.0904) radius 2.75
extrude "Stop screw head" add sketch "Stop screw head sketch" along normal blind 3 from surface at 0.5 separate body makes body 32 in component "Omni pivot"
sketch "Pivot tube sketch" plane through (0, 0, 0) normal (0, 1, 0) x (1, 0, 0) in component "Omni spring"
  circle A0 centre (24.0928, -42) radius 2.5
  circle A1 centre (24.0928, -42) radius 1.55
extrude "Pivot tube" add sketch "Pivot tube sketch" along normal blind 13.5 from surface at 7.5 separate body makes body 33 in component "Omni spring"
sketch "Spring coil sketch" plane through (0, 0, 0) normal (0, 1, 0) x (1, 0, 0) in component "Omni spring"
  circle A0 centre (24.0928, -42) radius 5.8
  circle A1 centre (24.0928, -42) radius 4.2
extrude "Spring coil" add sketch "Spring coil sketch" along normal blind 8.112 from surface at 8 separate body makes body 34 in component "Omni spring"
sketch "Spring rear leg sketch" plane through (0, 0, 0) normal (0, 1, 0) x (1, 0, 0) in component "Omni spring"
  line L0 (12.0928, -46.2) -> (19.4928, -46.2)
  line L1 (19.4928, -46.2) -> (19.4928, -47.8)
  line L2 (19.4928, -47.8) -> (12.0928, -47.8)
  line L3 (12.0928, -47.8) -> (12.0928, -46.2)
extrude "Spring rear leg" add sketch "Spring rear leg sketch" along normal blind 1.6 from surface at 8 separate body makes body 35 in component "Omni spring"
sketch "Spring arbor sketch" plane through (0, 0, 0) normal (0, 1, 0) x (1, 0, 0) in component "Omni spring"
  circle A0 centre (24.0928, -42) radius 3.7
  circle A1 centre (24.0928, -42) radius 2.6
extrude "Spring arbor" add sketch "Spring arbor sketch" along normal blind 9 from surface at 7.5 separate body makes body 36 in component "Omni spring"
sketch "Adjuster screw head sketch" plane through (0, 0, 0) normal (0, 0, 1) x (1, 0, 0) in component "Omni adjuster"
  line L0 (17.2728, 8.8) -> (15.6828, 11.554)
  line L1 (15.6828, 11.554) -> (12.5028, 11.554)
  line L2 (12.5028, 11.554) -> (10.9128, 8.8)
  line L3 (10.9128, 8.8) -> (12.5028, 6.046)
  line L4 (12.5028, 6.046) -> (15.6828, 6.046)
  line L5 (15.6828, 6.046) -> (17.2728, 8.8)
extrude "Adjuster screw head" add sketch "Adjuster screw head sketch" along normal blind 2 from surface at 44.2 separate body makes body 37 in component "Omni adjuster"
sketch "Adjuster screw sketch" plane through (0, 0, 0) normal (0, 0, 1) x (1, 0, 0) in component "Omni adjuster"
  circle A0 centre (14.0928, 8.8) radius 1.5
extrude "Adjuster screw" add sketch "Adjuster screw sketch" along normal blind 6 from surface at 38.2 separate body makes body 38 in component "Omni adjuster"
sketch "Rear nub sketch" plane through (0, 0, 0) normal (0, 0, 1) x (1, 0, 0) in component "Rear nub"
  circle A0 centre (-80, 0) radius 4
extrude "Rear nub" add sketch "Rear nub sketch" along normal blind 26 from surface at 20 separate body makes body 39 in component "Rear nub"
sketch "Seat on chamfer sketch" plane through (0, 0, 0) normal (0, 1, 0) x (1, 0, 0) in component "Rear nub"
  line L0 (-65, -35) -> (-112, -56.15)
  line L1 (-112, -56.15) -> (-112, -70)
  line L2 (-112, -70) -> (-65, -70)
  line L3 (-65, -70) -> (-65, -35)
extrude "Seat on chamfer" cut sketch "Seat on chamfer sketch" along normal blind 20 from surface at -10 bodies 39 in component "Rear nub"
sketch "Bumper plate L sketch" plane through (0, 0, 0) normal (0, 0, 1) x (1, 0, 0) in component "Bumper L"
  arc A0 (107.5962, 22.8703) -> (58.2911, 93.2853) centre (0, 0) ccw
  line L0 (58.2911, 93.2853) -> (56.9663, 91.1652)
  arc A1 (105.1509, 22.3505) -> (56.9663, 91.1652) centre (0, 0) ccw
  line L1 (105.1509, 22.3505) -> (107.5962, 22.8703)
extrude "Bumper plate L" add sketch "Bumper plate L sketch" along normal blind 25 from surface at 40 separate body makes body 40 in component "Bumper L"
sketch "Microswitch L sketch" plane through (0, 0, 0) normal (0, 0, 1) x (1, 0, 0) in component "Bumper switch L"
  line L0 (98.5442, 22.2509) -> (104.8511, 23.8234)
  line L1 (104.8511, 23.8234) -> (103.7625, 28.1898)
  line L2 (103.7625, 28.1898) -> (97.4555, 26.6173)
  line L3 (97.4555, 26.6173) -> (98.5442, 22.2509)
extrude "Microswitch L" add sketch "Microswitch L sketch" along normal blind 10 from surface at 47.5 separate body makes body 41 in component "Bumper switch L"
sketch "Bumper plate R sketch" plane through (0, 0, 0) normal (0, 0, 1) x (1, 0, 0) in component "Bumper R"
  arc A0 (58.2911, -93.2853) -> (107.5962, -22.8703) centre (0, 0) ccw
  line L0 (107.5962, -22.8703) -> (105.1509, -22.3505)
  arc A1 (56.9663, -91.1652) -> (105.1509, -22.3505) centre (0, 0) ccw
  line L1 (56.9663, -91.1652) -> (58.2911, -93.2853)
extrude "Bumper plate R" add sketch "Bumper plate R sketch" along normal blind 25 from surface at 40 separate body makes body 42 in component "Bumper R"
sketch "Microswitch R sketch" plane through (0, 0, 0) normal (0, 0, 1) x (1, 0, 0) in component "Bumper switch R"
  line L0 (97.4555, -26.6173) -> (103.7625, -28.1898)
  line L1 (103.7625, -28.1898) -> (104.8511, -23.8234)
  line L2 (104.8511, -23.8234) -> (98.5442, -22.2509)
  line L3 (98.5442, -22.2509) -> (97.4555, -26.6173)
extrude "Microswitch R" add sketch "Microswitch R sketch" along normal blind 10 from surface at 47.5 separate body makes body 43 in component "Bumper switch R"
sketch "Frame ring sketch" plane through (0, 0, 0) normal (0, 0, 1) x (1, 0, 0) in component "Upper frame"
  circle A0 centre (0, 0) radius 105
  circle A1 centre (0, 0) radius 90
extrude "Frame ring" add sketch "Frame ring sketch" along normal blind 30 from surface at 87 separate body makes body 44 in component "Upper frame"
sketch "Bridge web sketch" plane through (0, 0, 0) normal (0, 0, 1) x (1, 0, 0) in component "Upper frame"
  line L0 (32, -12.5) -> (92, -12.5)
  line L1 (92, -12.5) -> (92, 12.5)
  line L2 (92, 12.5) -> (32, 12.5)
  line L3 (32, 12.5) -> (32, -12.5)
extrude "Bridge web" add sketch "Bridge web sketch" along normal blind 3 from surface at 87 bodies 44 in component "Upper frame"
sketch "Bridge rib sketch" plane through (0, 0, 0) normal (0, 0, 1) x (1, 0, 0) in component "Upper frame"
  line L0 (32.5, -5) -> (90.5, -5)
  line L1 (90.5, -5) -> (90.5, 5)
  line L2 (90.5, 5) -> (32.5, 5)
  line L3 (32.5, 5) -> (32.5, -5)
extrude "Bridge rib" add sketch "Bridge rib sketch" along normal blind 8.5 from surface at 89.5 bodies 44 in component "Upper frame"
sketch "Spoke web sketch" plane through (0, 0, 0) normal (0, 0, 1) x (1, 0, 0) in component "Upper frame"
  line L0 (-92, -10) -> (-72, -10)
  line L1 (-72, -10) -> (-72, 10)
  line L2 (-72, 10) -> (-92, 10)
  line L3 (-92, 10) -> (-92, -10)
extrude "Spoke web" add sketch "Spoke web sketch" along normal blind 3 from surface at 87 bodies 44 in component "Upper frame"
sketch "Spoke rib sketch" plane through (0, 0, 0) normal (0, 0, 1) x (1, 0, 0) in component "Upper frame"
  line L0 (-92, -5) -> (-79, -5)
  line L1 (-79, -5) -> (-79, 5)
  line L2 (-79, 5) -> (-92, 5)
  line L3 (-92, 5) -> (-92, -5)
extrude "Spoke rib" add sketch "Spoke rib sketch" along normal blind 5.5 from surface at 89.5 bodies 44 in component "Upper frame"
sketch "Control deck sketch" plane through (0, 0, 0) normal (0, 0, 1) x (1, 0, 0) in component "Upper frame"
  line L0 (52, -12.5) -> (91.5, -12.5)
  line L1 (91.5, -12.5) -> (91.5, 36)
  line L2 (91.5, 36) -> (52, 36)
  line L3 (52, 36) -> (52, -12.5)
extrude "Control deck" add sketch "Control deck sketch" along normal blind 3 from surface at 87 bodies 44 in component "Upper frame"
sketch "Handle post sketch" plane through (0, 0, 0) normal (0, 0, 1) x (1, 0, 0) in component "Upper frame"
  line L0 (33, -7) -> (47, -7)
  line L1 (47, -7) -> (47, 7)
  line L2 (47, 7) -> (33, 7)
  line L3 (33, 7) -> (33, -7)
extrude "Handle post" add sketch "Handle post sketch" along normal blind 43 from surface at 97 bodies 44 in component "Upper frame"
sketch "ToF block F sketch" plane through (0, 0, 0) normal (0, 0, 1) x (1, 0, 0) in component "Upper frame"
  line L0 (88.1, -12.19) -> (101.1, -12.19)
  line L1 (101.1, -12.19) -> (101.1, 12.19)
  line L2 (101.1, 12.19) -> (88.1, 12.19)
  line L3 (88.1, 12.19) -> (88.1, -12.19)
extrude "ToF block F" add sketch "ToF block F sketch" along normal blind 30 from surface at 87 bodies 44 in component "Upper frame"